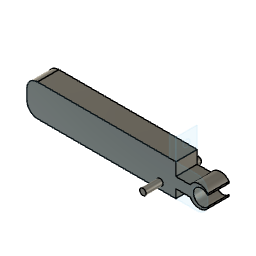
ian_use_this_file_2 (Autodesk Fusion 360 design; units mm, degrees)
Autodesk Fusion 360 part; units mm, degrees
note: some values were not read from the file. Chosen so that the rebuilt part matches the saved one: which bodies a step acts on.
sketch "Sketch1" plane through (0, 0, 0) normal (0, 1, 0) x (1, 0, 0)
  line L0 (0, 0) -> (85, 0)
  line L1 (85, 0) -> (85, -15)
  line L2 (85, -15) -> (0, -15)
  line L3 (0, -15) -> (0, 0)
  dimension "d1" = 85
  dimension "d2" = 15
  constraint horizontal L0
  constraint vertical L1
  constraint horizontal L2
  constraint vertical L3
  constraint coincident L0.start L3.end
  measures "d1" distance of L0.start L0.end
  measures "d2" distance of L0.start L2.end
extrude "Extrude1" add sketch "Sketch1" along normal blind 10 makes body 1
fillet "Fillet1" radius 5 4 edges at (0, 5, 15) (0, 5, 0) (85, 5, 15) (85, 5, 0) on bodies 1
sketch "Sketch2" plane through (0, 0, 15) normal (0, 0, 1) x (-1, 0, 0)
  line L0 (-80, 0) -> (-80, -10)
  line L1 (-80, -10) -> (-5, -10)
  line L2 (-5, -10) -> (-5, 0)
  line L3 (-5, 0) -> (-80, 0)
  line L4 (-67, -10) -> (-70, -10)
  line L5 (-70, -10) -> (-70, 0)
  line L6 (-70, 0) -> (-67, 0)
  line L7 (-67, 0) -> (-67, -10)
  dimension "d7" = 3
  dimension "d8" = 10
  constraint horizontal L4
  constraint vertical L5
  constraint horizontal L6
  constraint vertical L7
  constraint coincident L1 L4.start
  measures "d7" distance of L4.start L4.end
  measures "d8" distance of L0 L5
extrude "Extrude2" add sketch "Sketch2" along normal blind 10 contours L1 L3 L4 L5 L6 L7 bodies 1
sketch "Sketch3" plane through (0, 0, 0) normal (0, -1, 0) x (1, 0, 0)
  arc A0 (80, 0) -> (85, 5) centre (80, 5) ccw
  line L0 (85, 5) -> (85, 10)
  arc A1 (85, 10) -> (80, 15) centre (80, 10) ccw
  line L1 (80, 15) -> (70, 15)
  line L2 (70, 15) -> (70, 25)
  line L3 (70, 25) -> (67, 25)
  line L4 (67, 25) -> (67, 15)
  line L5 (67, 15) -> (5, 15)
  arc A2 (5, 15) -> (0, 10) centre (5, 10) ccw
  line L6 (0, 10) -> (0, 5)
  arc A3 (0, 5) -> (5, 0) centre (5, 5) ccw
  line L7 (5, 0) -> (80, 0)
  circle A4 centre (80, 7.4726) radius 2
  dimension "d11" = 4
  measures "d11" diameter of A4
extrude "Extrude3" cut sketch "Sketch3" against normal blind 13 contours A4 bodies 1
sketch "Sketch4" plane through (70, 0, 0) normal (1, 0, 0) x (0, 1, 0)
  line L0 (0, 15) -> (10, 15)
  line L1 (10, 15) -> (10, 25)
  line L2 (10, 25) -> (0, 25)
  line L3 (0, 25) -> (0, 15)
  circle A0 centre (5, 20.0248) radius 1.625
  dimension "d14" = 3.25
  measures "d14" diameter of A0
extrude "Extrude4" cut sketch "Sketch4" against normal blind 56 contours A0 bodies 1
sketch "Sketch5" plane through (0, 0, 0) normal (0, -1, 0) x (1, 0, 0)
  circle A0 centre (80, 7.4726) radius 2
  arc A1 (80, 0) -> (85, 5) centre (80, 5) ccw
  line L0 (85, 5) -> (85, 10)
  arc A2 (85, 10) -> (80, 15) centre (80, 10) ccw
  line L1 (80, 15) -> (70, 15)
  line L2 (70, 15) -> (70, 25)
  line L3 (70, 25) -> (67, 25)
  line L4 (67, 25) -> (67, 15)
  line L5 (67, 15) -> (5, 15)
  arc A3 (5, 15) -> (0, 10) centre (5, 10) ccw
  line L6 (0, 10) -> (0, 5)
  arc A4 (0, 5) -> (5, 0) centre (5, 5) ccw
  line L7 (5, 0) -> (80, 0)
sketch "Sketch6" plane through (70, 0, 0) normal (1, 0, 0) x (0, 1, 0)
  circle A0 centre (5, 20.0248) radius 1.625
  line L0 (0, 15) -> (10, 15)
  line L1 (10, 15) -> (10, 25)
  line L2 (10, 25) -> (0, 25)
  line L3 (0, 25) -> (0, 15)
sketch "Sketch7" plane through (85, 0, 0) normal (1, 0, 0) x (0, 1, 0)
  line L0 (0, 5) -> (10, 5)
  line L1 (10, 5) -> (10, 10)
  line L2 (10, 10) -> (0, 10)
  line L3 (0, 10) -> (0, 5)
  line L4 (0, 15) -> (10, 15)
  line L5 (10, 15) -> (10, 0)
  line L6 (10, 0) -> (0, 0)
  line L7 (0, 0) -> (0, 15)
  constraint horizontal L4
  constraint vertical L5
  constraint horizontal L6
  constraint vertical L7
extrude "Extrude5" cut sketch "Sketch7" against normal blind 15 bodies 1
sketch "Sketch8" plane through (70, 0, 0) normal (1, 0, 0) x (0, 1, 0)
  circle A0 centre (5, 20.0248) radius 1.625
  line L0 (10, 0) -> (10, 25)
  line L1 (10, 25) -> (0, 25)
  line L2 (0, 25) -> (0, 0)
  line L3 (0, 0) -> (10, 0)
  line L4 (0, 9) -> (10, 9)
  line L5 (10, 9) -> (10, 4)
  line L6 (10, 4) -> (0, 4)
  line L7 (0, 4) -> (0, 9)
  line L8 (10, 25) -> (0, 25)
  dimension "d19" = 5
  dimension "d20" = 10
  dimension "d21" = 16
  constraint horizontal L4
  constraint vertical L5
  constraint horizontal L6
  constraint vertical L7
  constraint coincident L2 L4.start
  measures "d19" distance of L4.start L6.end
  measures "d20" distance of L4.start L4.end
  measures "d21" distance of L4 L8
extrude "Extrude6" add sketch "Sketch8" along normal blind 7.5 contours L0 L2 L4 L5 L6 L7 bodies 1
cylinder "CylinderPrimitive1" add diameter 10 height -10 placed x (1, 0, 0) y (0, 0, -1) z (0, 1, 0) at (81.0326, 10, 6.5) separate body makes body 2
ref_plane "WorkPlane1" through (87, 0, 0) normal (1, 0, 0) x (0, 1, 0)
sketch "Sketch11" plane through (87, 0, 0) normal (1, 0, 0) x (0, 1, 0)
  line L0 (-1.0999, 12.5133) -> (11, 12.5133)
  line L1 (11, 12.5133) -> (11, 1)
  line L2 (11, 1) -> (-1.0999, 1)
  line L3 (-1.0999, 1) -> (-1.0999, 12.5133)
  constraint horizontal L0
  constraint vertical L1
  constraint horizontal L2
  constraint vertical L3
extrude "Extrude7" cut sketch "Sketch11" against normal blind 2 bodies 2
copy_body "CopyPasteBodies1" bodies 2 makes body 3
move_body "Move1" bodies 3 to x (1, 0, 0) y (0, 1, 0) z (0, 0, 1) at (19, 0, 0)
scale "Scale1" factors (0.75, 1, 0.75) about (104, 0, 3.457) bodies 3
move_body "Move2" bodies 3 to x (1, 0, 0) y (0, 1, 0) z (0, 0, 1) at (-19, 0, 0.7608)
combine "Combine1" operation add target body 1 tool bodies 2
split "Split1" by bodies 3 bodies 1 makes body 4 at (47.3333, 10, 5)
move_body "Move3" bodies 1 to x (1, 0, 0) y (0, 1, 0) z (0, 0, 1) at (20, 0, 0)
sketch "Sketch12" plane through (0, 0, 0) normal (0, -1, 0) x (1, 0, 0)
sketch "Sketch15" plane through (67, 0, 0) normal (-1, 0, 0) x (0, -1, 0)
  circle A0 centre (-5, 20.0248) radius 1.625
  line L0 (-10, 15) -> (0, 15)
  line L1 (0, 15) -> (0, 25)
  line L2 (0, 25) -> (-10, 25)
  line L3 (-10, 25) -> (-10, 15)
  line L4 (-10, 25) -> (0, 25)
  line L5 (0, 25) -> (0, 15)
  line L6 (0, 15) -> (-10, 15)
  line L7 (-10, 15) -> (-10, 25)
  constraint horizontal L4
  constraint vertical L5
  constraint horizontal L6
  constraint vertical L7
  constraint coincident L0.end L1.start
  constraint coincident L2.end L3.start
extrude "Extrude8" cut sketch "Sketch15" against normal blind 10 bodies 4
sketch "Sketch16" plane through (0, 0, 0) normal (0, -1, 0) x (1, 0, 0)
  circle A0 centre (62.5, 3) radius 1.5
  line L0 (5, 0) -> (80, 0)
  line L1 (70, 0) -> (70, 4)
  dimension "d40" = 3
  dimension "d41" = 3
  dimension "d42" = 7.5
  measures "d40" diameter of A0
  measures "d41" distance of A0.centre L0
  measures "d42" distance of A0.centre L1
extrude "Extrude9" add sketch "Sketch16" along normal blind 5 bodies 4
ref_plane "WorkPlane2" through (0, 5, 0) normal (0, 1, 0) x (0, 0, 1)
extrude "Extrude10" add 1 faces at (62.1279, -5, 3.2656) along direction (0, -1, 0) blind 3 on bodies 4 bodies 4
mirror "Mirror1" about plane through (0, 5, 0) normal (0, 1, 0) of "Extrude9", "Extrude10"
hidden bodies 1 3
